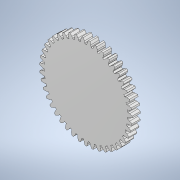
# Autodesk Inventor part: 最終段歯数43
Saved by Autodesk Inventor 2022.2 (Build 262287030, 287C)
## iProperties
Created: 2022-02-22
Part Number: 最終段歯数43
Material: Aluminum 2014-T6
Document SubType Name: Modeling
Designer: acps
Density: 2.78927 g/cm^3
Appearance: Satin
Author: acps
Autodesk Inventor part; units mm, degrees
ref_plane "YZ Plane" through (0, 0, 0) normal (1, 0, 0) x (0, 1, 0)
ref_plane "XZ Plane" through (0, 0, 0) normal (0, 1, 0) x (-1, 0, 0)
ref_plane "XY Plane" through (0, 0, 0) normal (0, 0, 1) x (1, 0, 0)
sketch "Sketch1" plane through (0, 0, 0) normal (0, 0, 1) x (1, 0, 0)
  arc A0 (0.499, 20.5965) -> (0.44, 20.2452) centre (3.1857, 19.9649) ccw
  arc A1 (0.7195, 21.3178) -> (0.499, 20.5965) centre (5.8188, 19.3641) ccw
  arc A2 (1.2603, 22.4647) -> (0.7195, 21.3178) centre (8.5494, 18.3267) ccw
  arc A3 (-2.5052, 20.4496) -> (-2.5124, 20.0935) centre (0.2448, 20.216) ccw
  arc A4 (-2.392, 21.1954) -> (-2.5052, 20.4496) centre (2.9373, 20.005) ccw
  arc A5 (-2.024, 22.4088) -> (-2.392, 21.1954) centre (5.7899, 19.3762) ccw
  arc A6 (-5.456, 19.867) -> (-5.4113, 19.5136) centre (-2.7013, 20.0362) ccw
  arc A7 (-5.4526, 20.6212) -> (-5.456, 19.867) centre (-0.0067, 20.2195) ccw
  arc A8 (-5.2652, 21.8753) -> (-5.4526, 20.6212) centre (2.907, 20.0127) ccw
  arc A9 (-8.2905, 18.8608) -> (-8.1948, 18.5178) centre (-5.5898, 19.4294) ccw
  arc A10 (-8.397, 19.6076) -> (-8.2905, 18.8608) centre (-2.9506, 20.003) ccw
  arc A11 (-8.3941, 20.8756) -> (-8.397, 19.6076) centre (-0.0379, 20.2227) ccw
  arc A12 (-10.9483, 17.4527) -> (-10.8037, 17.1272) centre (-8.3592, 18.4085) ccw
  arc A13 (-11.1624, 18.176) -> (-10.9483, 17.4527) centre (-5.8317, 19.3603) ccw
  arc A14 (-11.3442, 19.4309) -> (-11.1624, 18.176) centre (-2.9819, 20.0017) ccw
  arc A15 (-13.3728, 15.6727) -> (-13.1823, 15.3717) centre (-10.9504, 16.9952) ccw
  arc A16 (-13.6899, 16.3571) -> (-13.3728, 15.6727) centre (-8.5884, 18.3049) ccw
  arc A17 (-14.0524, 17.5721) -> (-13.6899, 16.3571) centre (-5.8624, 19.3543) ccw
  arc A18 (-15.5123, 13.5585) -> (-15.28, 13.2885) centre (-13.3082, 15.2197) ccw
  arc A19 (-15.9256, 14.1895) -> (-15.5123, 13.5585) centre (-11.1621, 16.8593) ccw
  arc A20 (-16.4612, 15.3388) -> (-15.9256, 14.1895) centre (-8.6179, 18.2945) ccw
  arc A21 (-17.3211, 11.1554) -> (-17.052, 10.9221) centre (-15.3824, 13.1198) ccw
  arc A22 (-17.8219, 11.7195) -> (-17.3211, 11.1554) centre (-13.4979, 15.0544) ccw
  arc A23 (-18.5191, 12.7786) -> (-17.8219, 11.7195) centre (-11.1898, 16.8448) ccw
  arc A24 (-18.7607, 8.5146) -> (-18.4605, 8.323) centre (-17.1287, 10.7403) ccw
  arc A25 (-19.3384, 8.9997) -> (-18.7607, 8.5146) centre (-15.546, 12.9287) ccw
  arc A26 (-20.1824, 9.946) -> (-19.3384, 8.9997) centre (-13.5232, 15.036) ccw
  arc A27 (-19.8006, 5.6923) -> (-19.4756, 5.5464) centre (-18.51, 8.1319) ccw
  arc A28 (-20.4426, 6.0881) -> (-19.8006, 5.6923) centre (-17.2627, 10.5274) ccw
  arc A29 (-21.4154, 6.9014) -> (-20.4426, 6.0881) centre (-15.5683, 12.9068) ccw
  arc A30 (-20.4184, 2.7486) -> (-20.0756, 2.6516) centre (-19.4967, 5.3501) ccw
  arc A31 (-21.1112, 3.0468) -> (-20.4184, 2.7486) centre (-18.6116, 7.9018) ccw
  arc A32 (-22.1921, 3.7098) -> (-21.1112, 3.0468) centre (-17.2817, 10.5025) ccw
  arc A33 (-20.601, -0.2536) -> (-20.2478, -0.2997) centre (-20.068, 2.4544) ccw
  arc A34 (-21.3299, -0.0595) -> (-20.601, -0.2536) centre (-19.5637, 5.1077) ccw
  arc A35 (-22.4957, 0.439) -> (-21.3299, -0.0595) centre (-18.6267, 7.8743) ccw
  arc A36 (-20.3445, -3.2504) -> (-19.9884, -3.2446) centre (-20.2115, -0.4937) ccw
  arc A37 (-21.0939, -3.1645) -> (-20.3445, -3.2504) centre (-20.0989, 2.2047) ccw
  arc A38 (-22.3199, -2.8411) -> (-21.0939, -3.1645) centre (-19.5747, 5.0784) ccw
  arc A39 (-19.6544, -6.178) -> (-19.3029, -6.1204) centre (-19.9242, -3.4312) ccw
  arc A40 (-20.4083, -6.2021) -> (-19.6544, -6.178) centre (-20.2058, -0.7452) ccw
  arc A41 (-21.6684, -6.0606) -> (-20.4083, -6.2021) centre (-20.1055, 2.1741) ccw
  arc A42 (-18.5455, -8.9738) -> (-18.2061, -8.8657) centre (-19.2123, -6.2957) ccw
  arc A43 (-19.2878, -9.1075) -> (-18.5455, -8.9738) centre (-19.8819, -3.6792) ccw
  arc A44 (-20.5551, -9.1509) -> (-19.2878, -9.1075) centre (-20.2078, -0.7764) ccw
  arc A45 (-17.0412, -11.5784) -> (-16.7212, -11.422) centre (-18.0909, -9.0259) ccw
  arc A46 (-17.7562, -11.8188) -> (-17.0412, -11.5784) centre (-19.1344, -6.5348) ccw
  arc A47 (-19.0036, -12.0463) -> (-17.7562, -11.8188) centre (-19.8794, -3.7104) ccw
  arc A48 (-15.1738, -13.9363) -> (-14.88, -13.7349) centre (-16.5839, -11.5638) ccw
  arc A49 (-15.8462, -14.2781) -> (-15.1738, -13.9363) centre (-17.979, -9.2512) ccw
  arc A50 (-17.0472, -14.6848) -> (-15.8462, -14.2781) centre (-19.1273, -6.5653) ccw
  arc A51 (-12.983, -15.9971) -> (-12.7216, -15.7551) centre (-14.7235, -13.8552) ccw
  arc A52 (-13.5984, -16.4332) -> (-12.983, -15.9971) centre (-16.4404, -11.7704) ccw
  arc A53 (-14.7274, -17.0104) -> (-13.5984, -16.4332) centre (-17.9676, -9.2803) ccw
  arc A54 (-10.5154, -17.7169) -> (-10.2921, -17.4395) centre (-12.5493, -15.8513) ccw
  arc A55 (-11.0608, -18.238) -> (-10.5154, -17.7169) centre (-14.5514, -14.0387) ccw
  arc A56 (-12.0937, -18.9735) -> (-11.0608, -18.238) centre (-16.4249, -11.7975) ccw
  arc A57 (-7.8237, -19.0592) -> (-7.6432, -18.7522) centre (-10.1076, -17.5096) ccw
  arc A58 (-8.2874, -19.6541) -> (-7.8237, -19.0592) centre (-12.3523, -16.0078) ccw
  arc A59 (-9.2022, -20.5321) -> (-8.2874, -19.6541) centre (-14.5321, -14.0633) ccw
  arc A60 (-4.9653, -19.9952) -> (-4.8314, -19.6652) centre (-7.4504, -18.7946) ccw
  arc A61 (-5.3375, -20.6514) -> (-4.9653, -19.9952) centre (-9.8899, -17.6357) ccw
  arc A62 (-6.1147, -21.6532) -> (-5.3375, -20.6514) centre (-12.3296, -16.0293) ccw
  arc A63 (-2.0011, -20.5051) -> (-1.9166, -20.1591) centre (-4.6345, -19.6791) ccw
  arc A64 (-2.2737, -21.2084) -> (-2.0011, -20.5051) centre (-7.2167, -18.8877) ccw
  arc A65 (-2.8968, -22.3127) -> (-2.2737, -21.2084) centre (-9.8643, -17.6537) ccw
  arc A66 (1.0058, -20.578) -> (1.039, -20.2233) centre (-1.7198, -20.1442) ccw
  arc A67 (0.8385, -21.3135) -> (1.0058, -20.578) centre (-4.3898, -19.7372) ccw
  arc A68 (0.3829, -22.4967) -> (0.8385, -21.3135) centre (-7.1888, -18.9018) ccw
  arc A69 (3.9913, -20.2122) -> (3.9724, -19.8565) centre (1.2315, -20.18) ccw
  arc A70 (3.9328, -20.9642) -> (3.9913, -20.2122) centre (-1.4692, -20.166) ccw
  arc A71 (3.6543, -22.2013) -> (3.9328, -20.9642) centre (-4.3601, -19.7471) ccw
  arc A72 (6.8917, -19.4157) -> (6.8213, -19.0665) centre (4.1566, -19.7856) ccw
  arc A73 (6.9433, -20.1682) -> (6.8917, -19.4157) centre (1.4826, -20.1651) ccw
  arc A74 (6.8479, -21.4326) -> (6.9433, -20.1682) centre (-1.4384, -20.1715) ccw
  arc A75 (9.6452, -18.2053) -> (9.5247, -17.8702) centre (6.9931, -18.9695) ccw
  arc A76 (9.8058, -18.9423) -> (9.6452, -18.2053) centre (4.4029, -19.7343) ccw
  arc A77 (9.8955, -20.2071) -> (9.8058, -18.9423) centre (1.5139, -20.166) ccw
  arc A78 (12.1931, -16.607) -> (12.0251, -16.2929) centre (9.6806, -17.7492) ccw
  arc A79 (12.4594, -17.3127) -> (12.1931, -16.607) centre (7.2293, -18.8829) ccw
  arc A80 (12.7323, -18.551) -> (12.4594, -17.3127) centre (4.434, -19.7306) ccw
  arc A81 (14.4812, -14.6547) -> (14.2692, -14.3684) centre (12.1617, -16.1505) ccw
  arc A82 (14.8474, -15.3141) -> (14.4812, -14.6547) centre (9.9017, -17.6291) ccw
  arc A83 (15.2976, -16.4995) -> (14.8474, -15.3141) centre (7.2595, -18.8748) ccw
  arc A84 (16.4606, -12.39) -> (16.2092, -12.1377) centre (14.3837, -14.2076) ccw
  arc A85 (16.9189, -12.9891) -> (16.4606, -12.39) centre (12.363, -15.9996) ccw
  arc A86 (17.537, -14.0963) -> (16.9189, -12.9891) centre (9.9304, -17.6166) ccw
  arc A87 (18.0892, -9.8613) -> (17.8037, -9.6483) centre (16.299, -11.962) ccw
  arc A88 (18.6298, -10.3873) -> (18.0892, -9.8613) centre (14.5608, -14.029) ccw
  arc A89 (19.4025, -11.3927) -> (18.6298, -10.3873) centre (12.3895, -15.983) ccw
  arc A90 (19.3322, -7.1224) -> (19.0188, -6.9532) centre (17.867, -9.4613) ccw
  arc A91 (19.9437, -7.5641) -> (19.3322, -7.1224) centre (16.4482, -11.7594) ccw
  arc A92 (20.8545, -8.4462) -> (19.9437, -7.5641) centre (14.5847, -14.0088) ccw
  arc A93 (20.1632, -4.2317) -> (19.8285, -4.11) centre (19.0542, -6.759) ccw
  arc A94 (20.8325, -4.5797) -> (20.1632, -4.2317) centre (17.9851, -9.2392) ccw
  arc A95 (21.8621, -5.3198) -> (20.8325, -4.5797) centre (16.4689, -11.7359) ccw
  arc A96 (20.5645, -1.2509) -> (20.2156, -1.1791) centre (19.8353, -3.9127) ccw
  arc A97 (21.2773, -1.4976) -> (20.5645, -1.2509) centre (19.1387, -6.5221) ccw
  arc A98 (22.4037, -2.0799) -> (21.2773, -1.4976) centre (18.0022, -9.213) ccw
  arc A99 (20.5275, 1.7567) -> (20.1719, 1.7769) centre (20.1936, -0.983) ccw
  arc A100 (21.2686, 1.6163) -> (20.5275, 1.7567) centre (19.8844, -3.666) ccw
  arc A101 (22.4678, 1.2042) -> (21.2686, 1.6163) centre (19.1518, -6.4937) ccw
  arc A102 (20.053, 4.7268) -> (19.6982, 4.695) centre (20.1215, 1.9677) ccw
  arc A103 (20.8066, 4.6959) -> (20.053, 4.7268) centre (20.2063, -0.7317) ccw
  arc A104 (22.053, 4.4627) -> (20.8066, 4.6959) centre (19.8932, -3.6359) ccw
  arc A105 (19.151, 7.5962) -> (18.8047, 7.513) centre (19.6206, 4.8765) ccw
  arc A106 (19.9012, 7.6753) -> (19.151, 7.5962) centre (20.0975, 2.2181) ccw
  arc A107 (21.1682, 7.6261) -> (19.9012, 7.6753) centre (20.2106, -0.7007) ccw
  arc A108 (17.8409, 10.3036) -> (17.5104, 10.171) centre (18.7015, 7.6813) ccw
  arc A109 (18.5716, 10.4911) -> (17.8409, 10.3036) centre (19.5603, 5.1207) ccw
  arc A110 (19.8322, 10.6269) -> (18.5716, 10.4911) centre (20.0972, 2.2494) ccw
  arc A111 (16.1506, 12.7915) -> (15.8429, 12.6121) centre (17.3838, 10.3224) ccw
  arc A112 (16.8461, 13.0834) -> (16.1506, 12.7915) centre (18.6063, 7.9141) ccw
  arc A113 (18.0736, 13.4013) -> (16.8461, 13.0834) centre (19.5555, 5.1516) ccw
  arc A114 (14.116, 15.0067) -> (13.8377, 14.7845) centre (15.6956, 12.7435) ccw
  arc A115 (14.7617, 15.3968) -> (14.116, 15.0067) centre (17.2557, 10.5389) ccw
  arc A116 (15.9298, 15.89) -> (14.7617, 15.3968) centre (18.597, 7.944) ccw
  arc A117 (11.7806, 16.9021) -> (11.5376, 16.6417) centre (13.6728, 14.893) ccw
  arc A118 (12.3626, 17.382) -> (11.7806, 16.9021) centre (15.5374, 12.939) ccw
  arc A119 (13.4464, 18.0401) -> (12.3626, 17.382) centre (17.2422, 10.5671) ccw
  arc A120 (9.1941, 18.4373) -> (8.9916, 18.1442) centre (11.3587, 16.725) ccw
  arc A121 (9.6891, 18.9862) -> (9.1941, 18.4373) centre (13.4878, 15.0634) ccw
  arc A122 (10.6764, 19.8056) -> (9.6891, 18.9862) centre (15.5198, 12.965) ccw
  arc A123 (6.4116, 19.5795) -> (6.254, 19.2601) centre (8.8025, 18.2006) ccw
  arc A124 (6.8307, 20.2066) -> (6.4116, 19.5795) centre (11.1509, 16.8667) ccw
  arc A125 (7.6789, 21.1491) -> (6.8307, 20.2066) centre (13.4668, 15.0866) ccw
  arc A126 (3.4925, 20.3043) -> (3.383, 19.9654) centre (6.0586, 19.2883) ccw
  arc A127 (3.8084, 20.9726) -> (3.4925, 20.3043) centre (8.5762, 18.3106) ccw
  arc A128 (4.5178, 22.0418) -> (3.8084, 20.9726) centre (11.1266, 16.8865) ccw
  arc A129 (-0.44, 20.2452) -> (-0.499, 20.5965) centre (-3.1857, 19.9649) ccw
  arc A130 (-0.499, 20.5965) -> (-0.7195, 21.3178) centre (-5.8188, 19.3641) ccw
  arc A131 (-0.7195, 21.3178) -> (-1.2603, 22.4647) centre (-8.5494, 18.3267) ccw
  arc A132 (-3.383, 19.9654) -> (-3.4925, 20.3043) centre (-6.0586, 19.2883) ccw
  arc A133 (-3.4925, 20.3043) -> (-3.8158, 20.9859) centre (-8.5762, 18.3106) ccw
  arc A134 (-3.8158, 20.9859) -> (-4.5178, 22.0418) centre (-11.1266, 16.8866) ccw
  arc A135 (-6.254, 19.2601) -> (-6.4116, 19.5795) centre (-8.8025, 18.2006) ccw
  arc A136 (-6.4116, 19.5795) -> (-6.8307, 20.2066) centre (-11.1509, 16.8667) ccw
  arc A137 (-6.8307, 20.2066) -> (-7.6789, 21.1491) centre (-13.4668, 15.0866) ccw
  arc A138 (-8.9916, 18.1442) -> (-9.1941, 18.4373) centre (-11.3587, 16.725) ccw
  arc A139 (-9.1941, 18.4373) -> (-9.7, 18.9968) centre (-13.4878, 15.0634) ccw
  arc A140 (-9.7, 18.9968) -> (-10.6764, 19.8056) centre (-15.5199, 12.965) ccw
  arc A141 (-11.5376, 16.6417) -> (-11.7806, 16.9021) centre (-13.6728, 14.893) ccw
  arc A142 (-11.7806, 16.9021) -> (-12.3626, 17.382) centre (-15.5374, 12.939) ccw
  arc A143 (-12.3626, 17.382) -> (-13.4464, 18.0401) centre (-17.2422, 10.5671) ccw
  arc A144 (-13.8377, 14.7845) -> (-14.116, 15.0067) centre (-15.6956, 12.7435) ccw
  arc A145 (-14.116, 15.0067) -> (-14.7617, 15.3968) centre (-17.2557, 10.5389) ccw
  arc A146 (-14.7617, 15.3968) -> (-15.9298, 15.89) centre (-18.597, 7.944) ccw
  arc A147 (-15.8429, 12.6121) -> (-16.1506, 12.7915) centre (-17.3838, 10.3224) ccw
  arc A148 (-16.1506, 12.7915) -> (-16.8461, 13.0834) centre (-18.6063, 7.9141) ccw
  arc A149 (-16.8461, 13.0834) -> (-18.0736, 13.4013) centre (-19.5555, 5.1516) ccw
  arc A150 (-17.5104, 10.171) -> (-17.8409, 10.3036) centre (-18.7015, 7.6813) ccw
  arc A151 (-17.8409, 10.3036) -> (-18.5716, 10.4911) centre (-19.5603, 5.1207) ccw
  arc A152 (-18.5716, 10.4911) -> (-19.8322, 10.6269) centre (-20.0972, 2.2494) ccw
  arc A153 (-18.8047, 7.513) -> (-19.151, 7.5962) centre (-19.6206, 4.8765) ccw
  arc A154 (-19.151, 7.5962) -> (-19.9012, 7.6753) centre (-20.0975, 2.2181) ccw
  arc A155 (-19.9012, 7.6753) -> (-21.1682, 7.6261) centre (-20.2106, -0.7007) ccw
  arc A156 (-19.6982, 4.695) -> (-20.053, 4.7268) centre (-20.1215, 1.9677) ccw
  arc A157 (-20.053, 4.7268) -> (-20.8066, 4.6959) centre (-20.2063, -0.7317) ccw
  arc A158 (-20.8066, 4.6959) -> (-22.053, 4.4627) centre (-19.8932, -3.6359) ccw
  arc A159 (-20.1719, 1.7769) -> (-20.5275, 1.7567) centre (-20.1936, -0.983) ccw
  arc A160 (-20.5275, 1.7567) -> (-21.2686, 1.6163) centre (-19.8844, -3.666) ccw
  arc A161 (-21.2686, 1.6163) -> (-22.4678, 1.2042) centre (-19.1518, -6.4937) ccw
  arc A162 (-20.2156, -1.1791) -> (-20.5645, -1.2509) centre (-19.8353, -3.9127) ccw
  arc A163 (-20.5645, -1.2509) -> (-21.2773, -1.4976) centre (-19.1387, -6.5221) ccw
  arc A164 (-21.2773, -1.4976) -> (-22.4037, -2.0799) centre (-18.0022, -9.213) ccw
  arc A165 (-19.8285, -4.11) -> (-20.1632, -4.2317) centre (-19.0542, -6.759) ccw
  arc A166 (-20.1632, -4.2317) -> (-20.8325, -4.5797) centre (-17.9851, -9.2392) ccw
  arc A167 (-20.8325, -4.5797) -> (-21.8621, -5.3198) centre (-16.4689, -11.7359) ccw
  arc A168 (-19.0188, -6.9532) -> (-19.3322, -7.1224) centre (-17.867, -9.4613) ccw
  arc A169 (-19.3322, -7.1224) -> (-19.9437, -7.5641) centre (-16.4482, -11.7594) ccw
  arc A170 (-19.9437, -7.5641) -> (-20.8545, -8.4462) centre (-14.5847, -14.0088) ccw
  arc A171 (-17.8037, -9.6483) -> (-18.0892, -9.8613) centre (-16.299, -11.962) ccw
  arc A172 (-18.0892, -9.8613) -> (-18.6298, -10.3873) centre (-14.5608, -14.029) ccw
  arc A173 (-18.6298, -10.3873) -> (-19.4025, -11.3927) centre (-12.3895, -15.983) ccw
  arc A174 (-16.2092, -12.1377) -> (-16.4606, -12.39) centre (-14.3837, -14.2076) ccw
  arc A175 (-16.4606, -12.39) -> (-16.9189, -12.9891) centre (-12.363, -15.9996) ccw
  arc A176 (-16.9189, -12.9891) -> (-17.537, -14.0963) centre (-9.9304, -17.6166) ccw
  arc A177 (-14.2692, -14.3684) -> (-14.4812, -14.6547) centre (-12.1617, -16.1505) ccw
  arc A178 (-14.4812, -14.6547) -> (-14.8474, -15.3141) centre (-9.9017, -17.6291) ccw
  arc A179 (-14.8474, -15.3141) -> (-15.2976, -16.4995) centre (-7.2595, -18.8748) ccw
  arc A180 (-12.0251, -16.2929) -> (-12.1931, -16.607) centre (-9.6806, -17.7492) ccw
  arc A181 (-12.1931, -16.607) -> (-12.4594, -17.3127) centre (-7.2293, -18.8829) ccw
  arc A182 (-12.4594, -17.3127) -> (-12.7323, -18.551) centre (-4.434, -19.7306) ccw
  arc A183 (-9.5247, -17.8702) -> (-9.6452, -18.2053) centre (-6.9931, -18.9695) ccw
  arc A184 (-9.6452, -18.2053) -> (-9.8058, -18.9423) centre (-4.4029, -19.7343) ccw
  arc A185 (-9.8058, -18.9423) -> (-9.8955, -20.2071) centre (-1.5139, -20.166) ccw
  arc A186 (-6.8213, -19.0665) -> (-6.8917, -19.4157) centre (-4.1566, -19.7856) ccw
  arc A187 (-6.8917, -19.4157) -> (-6.9433, -20.1682) centre (-1.4826, -20.1651) ccw
  arc A188 (-6.9433, -20.1682) -> (-6.8479, -21.4326) centre (1.4384, -20.1715) ccw
  arc A189 (-3.9724, -19.8565) -> (-3.9913, -20.2122) centre (-1.2315, -20.18) ccw
  arc A190 (-3.9913, -20.2122) -> (-3.9328, -20.9642) centre (1.4692, -20.166) ccw
  arc A191 (-3.9328, -20.9642) -> (-3.6543, -22.2013) centre (4.3601, -19.7471) ccw
  arc A192 (-1.039, -20.2233) -> (-1.0058, -20.578) centre (1.7198, -20.1442) ccw
  arc A193 (-1.0058, -20.578) -> (-0.8385, -21.3135) centre (4.3898, -19.7372) ccw
  arc A194 (-0.8385, -21.3135) -> (-0.3829, -22.4967) centre (7.1888, -18.9018) ccw
  arc A195 (1.9166, -20.1591) -> (2.0011, -20.5051) centre (4.6345, -19.6791) ccw
  arc A196 (2.0011, -20.5051) -> (2.2737, -21.2084) centre (7.2167, -18.8877) ccw
  arc A197 (2.2737, -21.2084) -> (2.8968, -22.3127) centre (9.8643, -17.6537) ccw
  arc A198 (4.8314, -19.6652) -> (4.9653, -19.9952) centre (7.4504, -18.7946) ccw
  arc A199 (4.9653, -19.9952) -> (5.3375, -20.6514) centre (9.8899, -17.6357) ccw
  arc A200 (5.3375, -20.6514) -> (6.1147, -21.6532) centre (12.3296, -16.0293) ccw
  arc A201 (7.6432, -18.7522) -> (7.8237, -19.0592) centre (10.1076, -17.5096) ccw
  arc A202 (7.8237, -19.0592) -> (8.2874, -19.6541) centre (12.3523, -16.0078) ccw
  arc A203 (8.2874, -19.6541) -> (9.2022, -20.5321) centre (14.5321, -14.0633) ccw
  arc A204 (10.2921, -17.4395) -> (10.5154, -17.7169) centre (12.5493, -15.8513) ccw
  arc A205 (10.5154, -17.7169) -> (11.0608, -18.238) centre (14.5514, -14.0387) ccw
  arc A206 (11.0608, -18.238) -> (12.0937, -18.9735) centre (16.4249, -11.7975) ccw
  arc A207 (12.7216, -15.7551) -> (12.983, -15.9971) centre (14.7235, -13.8552) ccw
  arc A208 (12.983, -15.9971) -> (13.5984, -16.4332) centre (16.4404, -11.7704) ccw
  arc A209 (13.5984, -16.4332) -> (14.7274, -17.0104) centre (17.9676, -9.2803) ccw
  arc A210 (14.88, -13.7349) -> (15.1738, -13.9363) centre (16.5839, -11.5638) ccw
  arc A211 (15.1738, -13.9363) -> (15.8462, -14.2781) centre (17.979, -9.2512) ccw
  arc A212 (15.8462, -14.2781) -> (17.0472, -14.6848) centre (19.1273, -6.5653) ccw
  arc A213 (16.7212, -11.422) -> (17.0412, -11.5784) centre (18.0909, -9.0259) ccw
  arc A214 (17.0412, -11.5784) -> (17.7562, -11.8188) centre (19.1344, -6.5348) ccw
  arc A215 (17.7562, -11.8188) -> (19.0036, -12.0463) centre (19.8794, -3.7104) ccw
  arc A216 (18.2061, -8.8657) -> (18.5455, -8.9738) centre (19.2123, -6.2957) ccw
  arc A217 (18.5455, -8.9738) -> (19.2878, -9.1075) centre (19.8819, -3.6792) ccw
  arc A218 (19.2878, -9.1075) -> (20.5551, -9.1509) centre (20.2078, -0.7764) ccw
  arc A219 (19.3029, -6.1204) -> (19.6544, -6.178) centre (19.9242, -3.4312) ccw
  arc A220 (19.6544, -6.178) -> (20.4083, -6.2021) centre (20.2058, -0.7452) ccw
  arc A221 (20.4083, -6.2021) -> (21.6684, -6.0606) centre (20.1055, 2.1741) ccw
  arc A222 (19.9884, -3.2446) -> (20.3445, -3.2504) centre (20.2114, -0.4937) ccw
  arc A223 (20.3445, -3.2504) -> (21.079, -3.1673) centre (20.0989, 2.2048) ccw
  arc A224 (21.079, -3.1673) -> (22.3199, -2.8411) centre (19.5747, 5.0784) ccw
  arc A225 (20.2478, -0.2997) -> (20.601, -0.2536) centre (20.068, 2.4544) ccw
  arc A226 (20.601, -0.2536) -> (21.3299, -0.0595) centre (19.5637, 5.1077) ccw
  arc A227 (21.3299, -0.0595) -> (22.4957, 0.439) centre (18.6267, 7.8743) ccw
  arc A228 (20.0756, 2.6516) -> (20.4184, 2.7486) centre (19.4967, 5.3501) ccw
  arc A229 (20.4184, 2.7486) -> (21.1112, 3.0468) centre (18.6116, 7.9018) ccw
  arc A230 (21.1112, 3.0468) -> (22.1921, 3.7098) centre (17.2817, 10.5025) ccw
  arc A231 (19.4756, 5.5464) -> (19.8006, 5.6923) centre (18.51, 8.1319) ccw
  arc A232 (19.8006, 5.6923) -> (20.4426, 6.0881) centre (17.2627, 10.5274) ccw
  arc A233 (20.4426, 6.0881) -> (21.4154, 6.9014) centre (15.5683, 12.9068) ccw
  arc A234 (18.4605, 8.323) -> (18.7607, 8.5146) centre (17.1287, 10.7403) ccw
  arc A235 (18.7607, 8.5146) -> (19.3384, 8.9997) centre (15.546, 12.9287) ccw
  arc A236 (19.3384, 8.9997) -> (20.1824, 9.946) centre (13.5232, 15.036) ccw
  arc A237 (17.052, 10.9221) -> (17.3211, 11.1554) centre (15.3824, 13.1198) ccw
  arc A238 (17.3211, 11.1554) -> (17.8219, 11.7195) centre (13.4979, 15.0544) ccw
  arc A239 (17.8219, 11.7195) -> (18.5191, 12.7786) centre (11.1898, 16.8448) ccw
  arc A240 (15.28, 13.2885) -> (15.5123, 13.5585) centre (13.3082, 15.2197) ccw
  arc A241 (15.5123, 13.5585) -> (15.9256, 14.1895) centre (11.1621, 16.8593) ccw
  arc A242 (15.9256, 14.1895) -> (16.4612, 15.3388) centre (8.6179, 18.2945) ccw
  arc A243 (13.1823, 15.3717) -> (13.3728, 15.6727) centre (10.9504, 16.9952) ccw
  arc A244 (13.3728, 15.6727) -> (13.6899, 16.3571) centre (8.5884, 18.3049) ccw
  arc A245 (13.6899, 16.3571) -> (14.0524, 17.5721) centre (5.8624, 19.3543) ccw
  arc A246 (10.8037, 17.1272) -> (10.9483, 17.4527) centre (8.3592, 18.4085) ccw
  arc A247 (10.9483, 17.4527) -> (11.1624, 18.176) centre (5.8317, 19.3603) ccw
  arc A248 (11.1624, 18.176) -> (11.3442, 19.4309) centre (2.9819, 20.0017) ccw
  arc A249 (8.1948, 18.5178) -> (8.2905, 18.8608) centre (5.5898, 19.4294) ccw
  arc A250 (8.2905, 18.8608) -> (8.397, 19.6076) centre (2.9506, 20.003) ccw
  arc A251 (8.397, 19.6076) -> (8.3941, 20.8756) centre (0.0379, 20.2227) ccw
  arc A252 (5.4113, 19.5136) -> (5.456, 19.867) centre (2.7013, 20.0362) ccw
  arc A253 (5.456, 19.867) -> (5.4537, 20.6061) centre (0.0067, 20.2195) ccw
  arc A254 (5.4537, 20.6061) -> (5.2652, 21.8753) centre (-2.907, 20.0127) ccw
  arc A255 (2.5124, 20.0935) -> (2.5052, 20.4496) centre (-0.2448, 20.216) ccw
  arc A256 (2.5052, 20.4496) -> (2.392, 21.1954) centre (-2.9373, 20.005) ccw
  arc A257 (2.392, 21.1954) -> (2.024, 22.4088) centre (-5.7899, 19.3762) ccw
  arc A258 (0.44, 20.2452) -> (-0.44, 20.2452) centre (0, 0) ccw
  arc A259 (-2.5124, 20.0935) -> (-3.383, 19.9654) centre (0, 0) ccw
  arc A260 (-5.4113, 19.5136) -> (-6.254, 19.2601) centre (0, 0) ccw
  arc A261 (-8.1948, 18.5178) -> (-8.9916, 18.1442) centre (0, 0) ccw
  arc A262 (-10.8037, 17.1272) -> (-11.5376, 16.6417) centre (0, 0) ccw
  arc A263 (-13.1823, 15.3717) -> (-13.8377, 14.7845) centre (0, 0) ccw
  arc A264 (-15.28, 13.2885) -> (-15.8429, 12.6121) centre (0, 0) ccw
  arc A265 (-17.052, 10.9221) -> (-17.5104, 10.171) centre (0, 0) ccw
  arc A266 (-18.4605, 8.323) -> (-18.8047, 7.513) centre (0, 0) ccw
  arc A267 (-19.4756, 5.5464) -> (-19.6982, 4.695) centre (0, 0) ccw
  arc A268 (-20.0756, 2.6516) -> (-20.1719, 1.7769) centre (0, 0) ccw
  arc A269 (-20.2478, -0.2997) -> (-20.2156, -1.1791) centre (0, 0) ccw
  arc A270 (-19.9884, -3.2446) -> (-19.8285, -4.11) centre (0, 0) ccw
  arc A271 (-19.3029, -6.1204) -> (-19.0188, -6.9532) centre (0, 0) ccw
  arc A272 (-18.2061, -8.8657) -> (-17.8037, -9.6483) centre (0, 0) ccw
  arc A273 (-16.7212, -11.422) -> (-16.2092, -12.1377) centre (0, 0) ccw
  arc A274 (-14.88, -13.7349) -> (-14.2692, -14.3684) centre (0, 0) ccw
  arc A275 (-12.7216, -15.7551) -> (-12.0251, -16.2929) centre (0, 0) ccw
  arc A276 (-10.2921, -17.4395) -> (-9.5247, -17.8702) centre (0, 0) ccw
  arc A277 (-7.6432, -18.7522) -> (-6.8213, -19.0665) centre (0, 0) ccw
  arc A278 (-4.8314, -19.6652) -> (-3.9724, -19.8565) centre (0, 0) ccw
  arc A279 (-1.9166, -20.1591) -> (-1.039, -20.2233) centre (0, 0) ccw
  arc A280 (1.039, -20.2233) -> (1.9166, -20.1591) centre (0, 0) ccw
  arc A281 (3.9724, -19.8565) -> (4.8314, -19.6652) centre (0, 0) ccw
  arc A282 (6.8213, -19.0665) -> (7.6432, -18.7522) centre (0, 0) ccw
  arc A283 (9.5247, -17.8702) -> (10.2921, -17.4395) centre (0, 0) ccw
  arc A284 (12.0251, -16.2929) -> (12.7216, -15.7551) centre (0, 0) ccw
  arc A285 (14.2692, -14.3684) -> (14.88, -13.7349) centre (0, 0) ccw
  arc A286 (16.2092, -12.1377) -> (16.7212, -11.422) centre (0, 0) ccw
  arc A287 (17.8037, -9.6483) -> (18.2061, -8.8657) centre (0, 0) ccw
  arc A288 (19.0188, -6.9532) -> (19.3029, -6.1204) centre (0, 0) ccw
  arc A289 (19.8285, -4.11) -> (19.9884, -3.2446) centre (0, 0) ccw
  arc A290 (20.2156, -1.1791) -> (20.2478, -0.2997) centre (0, 0) ccw
  arc A291 (20.1719, 1.7769) -> (20.0756, 2.6516) centre (0, 0) ccw
  arc A292 (19.6982, 4.695) -> (19.4756, 5.5464) centre (0, 0) ccw
  arc A293 (18.8047, 7.513) -> (18.4605, 8.323) centre (0, 0) ccw
  arc A294 (17.5104, 10.171) -> (17.052, 10.9221) centre (0, 0) ccw
  arc A295 (15.8429, 12.6121) -> (15.28, 13.2885) centre (0, 0) ccw
  arc A296 (13.8377, 14.7845) -> (13.1823, 15.3717) centre (0, 0) ccw
  arc A297 (11.5376, 16.6417) -> (10.8037, 17.1272) centre (0, 0) ccw
  arc A298 (8.9916, 18.1442) -> (8.1948, 18.5178) centre (0, 0) ccw
  arc A299 (6.254, 19.2601) -> (5.4113, 19.5136) centre (0, 0) ccw
  arc A300 (3.383, 19.9654) -> (2.5124, 20.0935) centre (0, 0) ccw
  arc A301 (-1.2603, 22.4647) -> (-2.024, 22.4088) centre (0, 0) ccw
  arc A302 (-4.5178, 22.0418) -> (-5.2652, 21.8753) centre (0, 0) ccw
  arc A303 (-7.6789, 21.1491) -> (-8.3941, 20.8756) centre (0, 0) ccw
  arc A304 (-10.6764, 19.8056) -> (-11.3442, 19.4309) centre (0, 0) ccw
  arc A305 (-13.4464, 18.0401) -> (-14.0524, 17.5721) centre (0, 0) ccw
  arc A306 (-15.9298, 15.89) -> (-16.4612, 15.3388) centre (0, 0) ccw
  arc A307 (-18.0736, 13.4013) -> (-18.5191, 12.7786) centre (0, 0) ccw
  arc A308 (-19.8322, 10.6269) -> (-20.1824, 9.946) centre (0, 0) ccw
  arc A309 (-21.1682, 7.6261) -> (-21.4154, 6.9014) centre (0, 0) ccw
  arc A310 (-22.053, 4.4627) -> (-22.1921, 3.7098) centre (0, 0) ccw
  arc A311 (-22.4678, 1.2042) -> (-22.4957, 0.439) centre (0, 0) ccw
  arc A312 (-22.4037, -2.0799) -> (-22.3199, -2.8411) centre (0, 0) ccw
  arc A313 (-21.8621, -5.3198) -> (-21.6684, -6.0606) centre (0, 0) ccw
  arc A314 (-20.8545, -8.4462) -> (-20.5551, -9.1509) centre (0, 0) ccw
  arc A315 (-19.4025, -11.3927) -> (-19.0036, -12.0463) centre (0, 0) ccw
  arc A316 (-17.537, -14.0963) -> (-17.0472, -14.6848) centre (0, 0) ccw
  arc A317 (-15.2976, -16.4995) -> (-14.7274, -17.0104) centre (0, 0) ccw
  arc A318 (-12.7323, -18.551) -> (-12.0937, -18.9735) centre (0, 0) ccw
  arc A319 (-9.8955, -20.2071) -> (-9.2022, -20.5321) centre (0, 0) ccw
  arc A320 (-6.8479, -21.4326) -> (-6.1147, -21.6532) centre (0, 0) ccw
  arc A321 (-3.6543, -22.2013) -> (-2.8968, -22.3127) centre (0, 0) ccw
  arc A322 (-0.3829, -22.4967) -> (0.3829, -22.4967) centre (0, 0) ccw
  arc A323 (2.8968, -22.3127) -> (3.6543, -22.2013) centre (0, 0) ccw
  arc A324 (6.1147, -21.6532) -> (6.8479, -21.4326) centre (0, 0) ccw
  arc A325 (9.2022, -20.5321) -> (9.8955, -20.2071) centre (0, 0) ccw
  arc A326 (12.0937, -18.9735) -> (12.7323, -18.551) centre (0, 0) ccw
  arc A327 (14.7274, -17.0104) -> (15.2976, -16.4995) centre (0, 0) ccw
  arc A328 (17.0472, -14.6848) -> (17.537, -14.0963) centre (0, 0) ccw
  arc A329 (19.0036, -12.0463) -> (19.4025, -11.3927) centre (0, 0) ccw
  arc A330 (20.5551, -9.1509) -> (20.8545, -8.4462) centre (0, 0) ccw
  arc A331 (21.6684, -6.0606) -> (21.8621, -5.3198) centre (0, 0) ccw
  arc A332 (22.3199, -2.8411) -> (22.4037, -2.0799) centre (0, 0) ccw
  arc A333 (22.4957, 0.439) -> (22.4678, 1.2042) centre (0, 0) ccw
  arc A334 (22.1921, 3.7098) -> (22.053, 4.4627) centre (0, 0) ccw
  arc A335 (21.4154, 6.9014) -> (21.1682, 7.6261) centre (0, 0) ccw
  arc A336 (20.1824, 9.946) -> (19.8322, 10.6269) centre (0, 0) ccw
  arc A337 (18.5191, 12.7786) -> (18.0736, 13.4013) centre (0, 0) ccw
  arc A338 (16.4612, 15.3388) -> (15.9298, 15.89) centre (0, 0) ccw
  arc A339 (14.0524, 17.5721) -> (13.4464, 18.0401) centre (0, 0) ccw
  arc A340 (11.3442, 19.4309) -> (10.6764, 19.8056) centre (0, 0) ccw
  arc A341 (8.3941, 20.8756) -> (7.6789, 21.1491) centre (0, 0) ccw
  arc A342 (5.2652, 21.8753) -> (4.5178, 22.0418) centre (0, 0) ccw
  arc A343 (2.024, 22.4088) -> (1.2603, 22.4647) centre (0, 0) ccw
  point P0 (0, 0)
  constraints: 516 point on circle, 258 centre point, 2 horizontal alignment, 256 other
extrude "Extrusion1" add sketch "Sketch1" against normal blind 4
body "Solid1"
